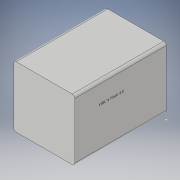
# Autodesk Inventor part: orca flash
Saved by Autodesk Inventor 2019 (Build 230136000, 136)
## iProperties
Created: 2019-03-06
Part Number: orca flash
Material: Generic
Document SubType Name: Modeling
Designer: Saumya
Density: 1 g/cm^3
Appearance: Default
Author: Saumya
Autodesk Inventor part; units mm, degrees
ref_plane "YZ Plane" through (0, 0, 0) normal (1, 0, 0) x (0, 1, 0)
ref_plane "XZ Plane" through (0, 0, 0) normal (0, 1, 0) x (-1, 0, 0)
ref_plane "XY Plane" through (0, 0, 0) normal (0, 0, 1) x (1, 0, 0)
sketch "Sketch1" plane through (0, 0, 0) normal (0, 0, 1) x (1, 0, 0)
  line L0 (19.688, 83.3096) -> (95.888, 83.3096)
  line L1 (95.888, 83.3096) -> (95.888, 7.1096)
  line L2 (95.888, 7.1096) -> (19.688, 7.1096)
  line L3 (19.688, 7.1096) -> (19.688, 83.3096)
  circle A0 centre (57.788, 45.2096) radius 23.0341
  point P0 (0, 0)
  dimension "d0" = 76.2
  dimension "d1" = 76.2
  constraints: 8 end point, 2 parallel, 1 centre point, 1 horizontal, 1 perpendicular
  measures "d0" distance of L1.end L2.end
  measures "d1" distance of L2.end L0.start
extrude "Extrusion1" add sketch "Sketch1" along normal blind 114.3 contours L0 L1 L2 L3 | A0
fillet "Fillet1" radius 3.175 4 edges at (19.688, 83.3096, 57.15) (95.888, 83.3096, 57.15) (95.888, 7.1096, 57.15) (19.688, 7.1096, 57.15)
sketch "Sketch2" plane through (95.888, 10.2846, 0) normal (1, 0, 0) x (0, 0, -1)
  line L0 (-83.9389, 49.2214) -> (-30.1471, 49.2214) construction
  line L1 (-30.1471, 49.2214) -> (-30.1471, 33.4582) construction
  line L2 (-30.1471, 33.4582) -> (-83.9389, 33.4582) construction
  line L3 (-83.9389, 33.4582) -> (-83.9389, 49.2214) construction
  point P0 (0, -10.2846)
  constraints: 2 other
sketch "Sketch3" plane through (0, 0, 0) normal (0, 0, -1) x (-1, 0, 0)
  circle A0 centre (-57.788, 45.2096) radius 18.2832
  line L0 (-92.713, 7.1096) -> (-22.863, 7.1096) projected
  line L1 (-95.888, 80.1346) -> (-95.888, 10.2846) projected
  point P0 (0, 0)
  dimension "d5" = 38.1
  dimension "d6" = 38.1
  constraints: 1 centre point
  measures "d5" distance from line of L0 A0.centre
  measures "d6" distance from line of L1 A0.centre
extrude "Extrusion2" cut sketch "Sketch3" against normal blind 7.62
body "Solid1"
